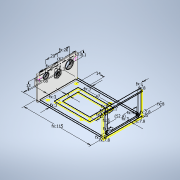
# Autodesk Inventor part: pi_shell_drill_guide_full
Saved by Autodesk Inventor 2022 (Build 260153000, 153)
## iProperties
Created: 2022-02-01
Part Number: pi_shell_drill_guide_full
Material: ABS Plastic
Document SubType Name: Modeling
Designer: Thomas
Density: 1.06 g/cm^3
Appearance: Smooth - White
Mass: 54.3446 g
Surface Area: 390.834 cm^2
Volume: 51.2684 cm^3
wall_thickness: 3.000 mm
outer_radius: 2.000 mm
inner_height: 38.000 mm
door_flange_thickness: 5.000 mm
m2p5_insert_top_diameter: 4.200 mm
insert_hole_angle: 8.00 deg
outer_width: 68.000 mm
outer_length: 115.000 mm
pcb_slide_thickness: 1.900 mm
Author: Thomas
Autodesk Inventor part; units mm, degrees
sketch "pi_base_plane" plane through (0, 0, 0) normal (0, 1, 0) x (-1, 0, 0)
  line L0 (0, 0) -> (115, 0)
  line L1 (115, 0) -> (115, 68)
  line L2 (115, 68) -> (0, 68)
  line L3 (0, 68) -> (0, 0)
  line L4 (3, 65) -> (112, 65)
  line L5 (112, 65) -> (112, 3)
  line L6 (112, 3) -> (3, 3)
  line L7 (3, 3) -> (3, 65)
  dimension "d0" = 115
  dimension "d1" = 68
  dimension "d2" = 3
  dimension "d3" = 3
  dimension "d4" = 3
  dimension "d5" = 3
  constraints: 16 end point, 4 parallel, 2 horizontal, 2 perpendicular
  measures "d0" distance of L2.end L1.end
  measures "d1" distance of L1.end L0.end
  measures "d2" distance between parallel lines of L4 L2
  measures "d3" distance between parallel lines of L1 L5
  measures "d4" distance between parallel lines of L0 L6
  measures "d5" distance between parallel lines of L3 L7
extrude "Extrusion1" add sketch "pi_base_plane" against normal blind 3 contours L3 L2 L1 L0 | L4 L5 L6 L7
extrude "Extrusion2" add sketch "pi_base_plane" along normal blind 38
sketch "pi_outline" plane through (0, 0, 0) normal (0, 1, 0) x (1, 0, 0)
  line L0 (-108, -6) -> (-23, -6)
  line L1 (-23, -6) -> (-23, -62)
  line L2 (-23, -62) -> (-108, -62)
  line L3 (-108, -62) -> (-108, -6)
  circle A0 centre (-104.5, -9.5) radius 1.35
  circle A1 centre (-104.5, -58.5) radius 1.35
  circle A2 centre (-46.5, -9.5) radius 1.35
  circle A3 centre (-46.5, -58.5) radius 1.35
  line L4 (-3, -65) -> (-112, -65) projected
  line L5 (-112, -3) -> (-3, -3) projected
  line L6 (-112, -65) -> (-112, -3) projected
  point P0 (0, 0)
  dimension "d10" = 56
  dimension "d11" = 85
  dimension "d12" = 2.7
  dimension "d13" = 3.5
  dimension "d14" = 3.5
  dimension "d15" = 2.7
  dimension "d16" = 3.5
  dimension "d17" = 3.5
  dimension "d18" = 2.7
  dimension "d19" = 3.5
  dimension "d20" = 58
  dimension "d21" = 2.7
  dimension "d22" = 3.5
  dimension "d23" = 58
  dimension "d24" = 62
  dimension "d25" = 3
  dimension "d26" = 4
  constraints: 8 end point, 4 centre point, 2 parallel, 1 horizontal, 1 perpendicular
  measures "d10" distance of L2.end L0.start
  measures "d11" distance between parallel lines of L1 L3
  measures "d12" diameter of A0
  measures "d13" distance from line of L0 A0.centre
  measures "d14" distance from line of A0.centre L3
  measures "d15" diameter of A1
  measures "d16" distance from line of L3 A1.centre
  measures "d17" distance from line of L2 A1.centre
  measures "d18" diameter of A2
  measures "d19" distance from line of A2.centre L0
  measures "d20" distance of A0.centre A2.centre
  measures "d21" diameter of A3
  measures "d22" distance from line of L2 A3.centre
  measures "d23" distance of A1.centre A3.centre
  measures "d24" distance between parallel lines of L4 L5
  measures "d25" distance between parallel lines of L0 L5
  measures "d26" distance between parallel lines of L3 L6
sketch "Sketch4" plane through (0, 0, 0) normal (0, 1, 0) x (1, 0, 0)
  circle A0 centre (-104.5, -9.5) radius 3.25
  circle A1 centre (-46.5, -9.5) radius 3.25
  circle A2 centre (-46.5, -58.5) radius 3.25
  circle A3 centre (-104.5, -58.5) radius 3.25
  point P0 (0, 0)
  dimension "d27" = 6.5
  dimension "d28" = 6.5
  dimension "d29" = 6.5
  dimension "d30" = 6.5
  constraints: 4 centre point, 4 coincident
  measures "d27" diameter of A0
  measures "d28" diameter of A3
  measures "d29" diameter of A1
  measures "d30" diameter of A2
extrude "Extrusion3" add sketch "Sketch4" along normal blind 0.4
sketch "Sketch5" plane through (-104.5, 0.4, 9.5) normal (0, 1, 0) x (1, 0, 0)
  circle A0 centre (0, 0) radius 3.25 projected
  circle A1 centre (0, 0) radius 2.1
  point P0 (104.5, 9.5)
  dimension "d34" = 4.2
  constraints: 1 centre point, 1 coincident
  measures "d34" diameter of A1
ref_plane "Work Plane1" through (-104.5, 0.4, 9.5) normal (0, 0, 1) x (1, 0, 0)
sketch "Sketch6" plane through (-104.5, 0.4, 9.5) normal (0, 0, 1) x (1, 0, 0)
  line L0 (3.25, 0) -> (-3.25, 0) projected
  line L1 (0, 0) -> (2.1, 0)
  line L2 (2.1, 0) -> (1.6222, -3.4)
  line L3 (-10.5, -3.4) -> (104.5, -3.4) projected
  line L4 (0, -3.4) -> (0, 0)
  line L5 (0, -3.4) -> (1.6222, -3.4)
  point P0 (104.5, -0.4)
  dimension "d35" = 2.1
  dimension "d36" = 82
  constraints: 8 end point, 3 point on line, 1 collinear, 1 midpoint, 1 perpendicular
  measures "d35" distance of L1.start L1.end
  measures "d36" angle of L0 L2
revolve "Revolution1" cut sketch "Sketch6" angle 360 about axis through (-104.5, -3, 9.5) along (0, 1, 0)
pattern_sketch "Sketch Driven Pattern1" of "Revolution1" from (-104.5, 0, 9.5) copies at (-46.5, 0, 9.5) at (-46.5, 0, 58.5) at (-104.5, 0, 58.5)
sketch "door" plane through (0, -3, 68) normal (1, 0, 0) x (0, 0, -1)
  line L0 (0, 41) -> (68, 41) projected
  line L1 (8, 41) -> (60, 41)
  line L2 (60, 41) -> (60, 13)
  line L3 (55, 8) -> (13, 8)
  line L4 (8, 13) -> (8, 41)
  line L5 (0, 0) -> (0, 41) projected
  line L6 (68, 0) -> (0, 0) projected
  line L7 (68, 0) -> (68, 41) projected
  arc A0 (55, 8) -> (60, 13) centre (55, 13) ccw
  arc A1 (8, 13) -> (13, 8) centre (13, 13) ccw
  line L8 (3, 46) -> (65, 46)
  line L9 (65, 46) -> (65, 13)
  arc A2 (55, 3) -> (65, 13) centre (55, 13) ccw
  line L10 (55, 3) -> (13, 3)
  arc A3 (3, 13) -> (13, 3) centre (13, 13) ccw
  line L11 (3, 13) -> (3, 46)
  line L12 (3, 41) -> (65, 41)
  line L13 (1, 41) -> (67, 41)
  line L14 (67, 41) -> (67, 39.1)
  line L15 (67, 39.1) -> (1, 39.1)
  line L16 (1, 39.1) -> (1, 41)
  line L17 (3, 3) -> (3, 41) projected
  line L18 (65, 41) -> (3, 41) projected
  line L19 (3, 41) -> (65, 41)
  line L20 (65, 41) -> (65, 41)
  line L21 (65, 41) -> (3, 41)
  line L22 (3, 41) -> (3, 41)
  point P0 (68, 3)
  point P1 (3, 41)
  point P2 (65, 41)
  point P3 (3, 41)
  point P4 (65, 41)
  dimension "d38" = 8
  dimension "d39" = 8
  dimension "d40" = 8
  dimension "d41" = 5
  dimension "d42" = 5
  dimension "d62" = 1
  dimension "d63" = 1
  dimension "d64" = 0
  dimension "d65" = 1.9
  constraints: 34 end point, 8 point on circle, 7 parallel, 4 centre point, 4 perpendicular, 4 tangent, 3 horizontal, 3 point on line, 1 collinear, 1 equal radius, 5 other
  measures "d38" distance between parallel lines of L4 L5
  measures "d39" distance between parallel lines of L3 L6
  measures "d40" distance between parallel lines of L7 L2
  measures "d41" radius of A0
  measures "d42" distance between parallel lines of L4 L11
  measures "d62" distance between parallel lines of L5 L16
  measures "d63" distance between parallel lines of L7 L14
  measures "d64" distance between parallel lines of L13 L0
  measures "d65" distance between parallel lines of L13 L15
extrude "door_cut" cut sketch "door" against normal blind 3 contours L0 L2 L15 L4 | L15 L2 A0 L3 A1 L4
extrude "Extrusion5" cut sketch "door" against normal blind 2 contours L0 L4 L15 L11 | L15 L4 A1 L3 A0 L2 L9 A2 L10 A3 L11 | L0 L9 L15 L2
sketch "Sketch8" plane through (-2, -3, 68) normal (1, 0, 0) x (0, 0, -1)
  circle A0 centre (7.8, 7.8) radius 2.1
  line L0 (0, 0) -> (0, 41) projected
  line L1 (68, 0) -> (0, 0) projected
  circle A1 centre (60.2, 7.8) radius 2.1
  line L2 (68, 0) -> (68, 41) projected
  point P0 (68, 3)
  dimension "d47" = 4.2
  dimension "d48" = 7.8
  dimension "d49" = 7.8
  dimension "d50" = 4.2
  dimension "d51" = 7.8
  dimension "d52" = 7.8
  dimension "d57" = 52.4
  constraints: 2 centre point
  measures "d47" diameter of A0
  measures "d48" distance from line of L0 A0.centre
  measures "d49" distance from line of A0.centre L1
  measures "d50" diameter of A1
  measures "d51" distance from line of L2 A1.centre
  measures "d52" distance from line of L1 A1.centre
  measures "d57" distance of A1.centre A0.centre
ref_plane "Work Plane2" through (-2, 4.8, 60.2) normal (0, 0, 1) x (1, 0, 0)
sketch "Sketch10" plane through (-3, 0, 3) normal (-1, 0, 0) x (0, 0, 1)
  arc A0 (52, 5) -> (57, 10) centre (52, 10) ccw projected
  arc A1 (52, 0) -> (62, 10) centre (52, 10) ccw projected
  line L0 (52, 5) -> (52, 0)
  line L1 (52, 0) -> (62, 0)
  line L2 (62, 0) -> (62, 10)
  line L3 (62, 10) -> (57, 10)
  arc A2 (5, 10) -> (10, 5) centre (10, 10) ccw projected
  line L4 (10, 5) -> (10, 0)
  arc A3 (0, 10) -> (10, 0) centre (10, 10) ccw projected
  line L5 (5, 10) -> (0, 10)
  line L6 (0, 10) -> (0, 0)
  line L7 (10, 0) -> (52, 0) projected
  line L8 (0, 0) -> (10, 0)
  point P0 (-3, 0)
  point P1 (57, 10)
  constraints: 16 end point, 5 perpendicular, 3 tangent, 2 vertical, 1 horizontal
extrude "Extrusion6" add sketch "Sketch10" along normal blind 3
sketch "Sketch9" plane through (-2, 4.8, 60.2) normal (0, 0, 1) x (1, 0, 0)
  line L0 (0, 0) -> (0, -2.0969)
  line L1 (0, -2.1) -> (0, 2.1) projected
  line L2 (-4, 5.2) -> (-4, 0.2) projected
  line L3 (-4, 0.2) -> (-4, -4.8) projected
  line L4 (-4, 5.2) -> (-4, -4.8) projected
  line L5 (0, 0) -> (0, -2.1)
  line L6 (0, -2.1) -> (-4, -1.5378)
  line L7 (-4, 0) -> (0, 0)
  line L8 (-4, -1.5378) -> (-4, 0)
  line L9 (-4, 0.2) -> (-4, -4.8) projected
  point P0 (2, -4.8)
  point P1 (-4, 0)
  point P2 (-4, -1.5378)
  dimension "d55" = 82
  constraints: 10 end point, 2 collinear, 2 point on line, 1 perpendicular, 1 vertical
  measures "d55" angle of L6 L0
revolve "Revolution2" cut sketch "Sketch9" angle 360 about axis through (-6, 4.8, 60.2) along (1, 0, 0)
ref_plane "Work Plane3" through (-2, 4.8, 7.8) normal (0, 0, -1) x (-1, 0, 0)
sketch "Sketch11" plane through (-2, 4.8, 7.8) normal (0, 0, -1) x (-1, 0, 0)
  line L0 (0, 2.1) -> (0, -2.1) projected
  line L1 (4, -4.8) -> (4, 5.2) projected
  line L2 (4, -4.8) -> (4, 0.2) projected
  line L3 (4, 0.2) -> (4, 5.2) projected
  line L4 (0, 0) -> (0, -2.1)
  line L5 (0, -2.1) -> (4, -1.5378)
  line L6 (4, -1.5378) -> (4, 0)
  line L7 (4, 0) -> (0, 0)
  point P0 (-2, -4.8)
  point P1 (4, 0)
  point P2 (4, -1.5378)
  dimension "d58" = 82
  constraints: 8 end point, 2 point on line, 1 collinear, 1 perpendicular
  measures "d58" angle of L0 L5
revolve "Revolution3" cut sketch "Sketch11" angle 360 about axis through (-6, 4.8, 7.8) along (1, 0, 0)
fillet "Fillet1" radius 1 6 edges at (-6, 10, 62.5) (-6, 6.4645, 58.5355) (-6, 2.5, 55) (-6, 2.5, 13) (-6, 6.4645, 9.4645) (-6, 10, 5.5)
fillet "Fillet2" radius 1 4 edges at (-49.75, 0, 58.5) (-107.75, 0, 58.5) (-49.75, 0, 9.5) (-107.75, 0, 9.5)
extrude "Extrusion7" cut sketch "door" against normal up to surface (112 mm away) contours L0 L11 L15 L16 | L0 L4 L15 L11 | L0 L2 L15 L4 | L0 L9 L15 L2 | L14 L15 L9 L0
sketch "Sketch12" plane through (-115, -3, 68) normal (0, 0, 1) x (1, 0, 0)
  line L0 (115, 39.1) -> (3, 39.1) projected
  circle A0 centre (20, 33) radius 1.325
  circle A1 centre (100, 33) radius 1.325
  line L1 (0, 0) -> (0, 41) projected
  line L2 (0, 41) -> (115, 41) projected
  line L3 (20, 33) -> (100, 33)
  point P0 (115, 3)
  dimension "d70" = 2.65
  dimension "d71" = 2.65
  dimension "d72" = 20
  dimension "d73" = 80
  dimension "d75" = 8
  constraints: 2 centre point, 2 end point, 1 horizontal
  measures "d70" diameter of A0
  measures "d71" diameter of A1
  measures "d72" distance from line of L1 L3.start
  measures "d73" distance of L3.end L3.start
  measures "d75" distance between parallel lines of L3 L2
extrude "M2.5 Side Fastners" cut sketch "Sketch12" against normal through all
sketch "Sketch14" plane through (-112, 0, 65) normal (1, 0, 0) x (0, 0, -1)
  line L0 (0, 36.1) -> (62, 36.1)
  circle A0 centre (31, 23.1) radius 3.15
  circle A1 centre (11, 30.1) radius 4.5
  circle A2 centre (51, 27) radius 6.5
  line L1 (36.5, 19.9246) -> (31, 16.7491)
  line L2 (31, 16.7491) -> (25.5, 19.9246)
  line L3 (25.5, 19.9246) -> (25.5, 26.2754)
  line L4 (25.5, 26.2754) -> (31, 29.4509)
  line L5 (31, 29.4509) -> (36.5, 26.2754)
  line L6 (36.5, 26.2754) -> (36.5, 19.9246)
  point P0 (65, 0)
  point P1 (0, 31)
  point P2 (62, 31)
  dimension "d78" = 6.3
  dimension "d79" = 9
  dimension "d80" = 13
  dimension "d81" = 6
  dimension "d82" = 9.1
  dimension "d84" = 62
  dimension "d85" = 31
  dimension "d90" = 11
  dimension "d93" = 13
  dimension "d94" = 20
  dimension "d95" = 20
  constraints: 14 end point, 3 centre point, 1 coincident, 1 horizontal, 1 vertical, 13 other
  measures "d78" diameter of A0
  measures "d79" diameter of A1
  measures "d80" diameter of A2
  measures "d81" vertical distance of A1.centre L0.start
  measures "d82" vertical distance of A2.centre L0.end
  measures "d84" distance of L0.end L0.start
  measures "d85" horizontal distance of A0.centre L0.start
  measures "d90" distance between parallel lines of L6 L3
  measures "d93" vertical distance of L0.start A0.centre
  measures "d94" horizontal distance of A0.centre A1.centre
  measures "d95" horizontal distance of A2.centre A0.centre
extrude "Connector and Mount Holes" cut sketch "Sketch14" against normal through all contours A0 | A1 | A2
extrude "Captive M6 Nut Indent" cut sketch "Sketch14" against normal blind 2 contours L1 L2 L3 L4 L5 L6
sketch "Sketch15" plane through (-115, -3, 0) normal (-1, 0, 0) x (0, 0, 1)
  line L0 (63.25, 30.75) -> (65.75, 30.75)
  line L1 (65.75, 30.75) -> (65.75, 19.75)
  line L2 (65.75, 19.75) -> (63.25, 19.75)
  line L3 (63.25, 19.75) -> (63.25, 30.75)
  line L4 (2.25, 30.75) -> (4.75, 30.75)
  line L5 (4.75, 30.75) -> (4.75, 19.75)
  line L6 (4.75, 19.75) -> (2.25, 19.75)
  line L7 (2.25, 19.75) -> (2.25, 30.75)
  line L8 (68, 0) -> (68, 41) projected
  line L9 (0, 41) -> (0, 0) projected
  circle A0 centre (34, 26.1) radius 3.15 projected
  point P0 (0, 3)
  dimension "d96" = 68
  dimension "d97" = 58.5
  dimension "d98" = 2.5
  dimension "d99" = 2.5
  dimension "d100" = 2.25
  dimension "d101" = 11
  dimension "d102" = 11
  dimension "d103" = 6.3
  dimension "d104" = 4.65
  dimension "d105" = 4.65
  constraints: 16 end point, 4 parallel, 2 horizontal, 2 perpendicular, 1 point on line
  measures "d96" distance between parallel lines of L8 L9
  measures "d97" distance between parallel lines of L3 L5
  measures "d98" distance between parallel lines of L5 L7
  measures "d99" distance between parallel lines of L1 L3
  measures "d100" distance between parallel lines of L7 L9
  measures "d101" distance between parallel lines of L4 L6
  measures "d102" distance of L0.end L1.end
  measures "d103" diameter of A0
  measures "d104" distance from line of A0.centre L4
  measures "d105" distance from line of A0.centre L0
extrude "Extrusion12" add sketch "Sketch15" along normal blind 5 contours L0 L1 L2 L3 | L4 L5 L6 L7
fillet "Fillet3" radius 5 2 edges at (-115, 16.75, 3.5) (-115, 16.75, 64.5)
sketch "Sketch16" plane through (0, 0, 0) normal (0, 1, 0) x (1, 0, 0)
  line L0 (-90.5, -47.5) -> (-43.5, -47.5)
  line L1 (-43.5, -47.5) -> (-43.5, -20.5)
  line L2 (-43.5, -20.5) -> (-90.5, -20.5)
  line L3 (-90.5, -20.5) -> (-90.5, -47.5)
  circle A0 centre (-104.5, -58.5) radius 2.1 projected
  circle A1 centre (-104.5, -9.5) radius 2.1 projected
  circle A2 centre (-46.5, -9.5) radius 2.1 projected
  circle A3 centre (-46.5, -58.5) radius 2.1 projected
  line L4 (-97.5, -54.5) -> (-36.5, -54.5)
  line L5 (-36.5, -54.5) -> (-36.5, -13.5)
  line L6 (-36.5, -13.5) -> (-97.5, -13.5)
  line L7 (-97.5, -13.5) -> (-97.5, -54.5)
  point P0 (0, 0)
  dimension "d109" = 47
  dimension "d110" = 27
  dimension "d111" = 14
  dimension "d112" = 11
  dimension "d113" = 7
  constraints: 16 end point, 4 parallel, 2 perpendicular, 1 horizontal, 3 other
  measures "d109" distance of L2.end L1.end
  measures "d110" distance of L1.end L0.end
  measures "d111" distance from line of A1.centre L3
  measures "d112" distance from line of L2 A2.centre
  measures "d113" distance between parallel lines of L3 L7
extrude "Extrusion13" cut sketch "Sketch16" against normal through all contours L3 L2 L1 L0
extrude "Extrusion14" cut sketch "Sketch16" against normal blind 2 contours L3 L2 L1 L0 | L7 L6 L5 L4
sketch "Sketch17" plane through (0, -2, 0) normal (0, 1, 0) x (1, 0, 0)
  circle A0 centre (-92.5, -49.5) radius 1.575
  line L0 (-36.5, -54.5) -> (-97.5, -54.5) projected
  line L1 (-90.5, -47.5) -> (-43.5, -47.5) projected
  line L2 (-97.5, -54.5) -> (-97.5, -13.5) projected
  circle A1 centre (-92.5, -18.5) radius 1.575
  line L3 (-97.5, -13.5) -> (-36.5, -13.5) projected
  circle A2 centre (-41.5, -49.5) radius 1.575
  line L4 (-36.5, -13.5) -> (-36.5, -54.5) projected
  circle A3 centre (-41.5, -18.5) radius 1.575
  line L5 (-90.5, -20.5) -> (-90.5, -47.5) projected
  line L6 (-90.5, -47.5) -> (-43.5, -47.5) projected
  point P0 (0, 0)
  point P1 (-90.5, -34)
  point P2 (-67, -47.5)
  dimension "d118" = 3.15
  dimension "d119" = 7
  dimension "d122" = 3.15
  dimension "d125" = 3.15
  dimension "d128" = 3.15
  dimension "d147" = 31
  dimension "d148" = 31
  dimension "d149" = 51
  dimension "d150" = 0
  dimension "d151" = 15.5
  dimension "d152" = 25.5
  dimension "d153" = 6
  dimension "d154" = 37
  constraints: 4 centre point, 2 midpoint
  measures "d118" diameter of A0
  measures "d119" distance between parallel lines of L0 L1
  measures "d122" diameter of A1
  measures "d125" diameter of A2
  measures "d128" diameter of A3
  measures "d147" distance of A2.centre A3.centre
  measures "d148" distance of A1.centre A0.centre
  measures "d149" distance of A2.centre A0.centre
  measures "d150" vertical distance of A3.centre A1.centre
  measures "d151" vertical distance of point (-90.5, -34) A0.centre
  measures "d152" horizontal distance of point (-67, -47.5) A0.centre
extrude "Extrusion15" cut sketch "Sketch17" against normal through all contours A0 | A1 | A2 | A3
sketch "Sketch18" plane through (0, 38, 0) normal (0, 1, 0) x (1, 0, 0)
  line L0 (-112, -65) -> (-113.5, -65)
  line L1 (-113.5, -65) -> (-113.5, -3)
  line L2 (-113.5, -3) -> (-112, -3)
  line L3 (-112, -3) -> (-112, -65)
  point P0 (0, 0)
  dimension "d133" = 1.5
  constraints: 8 end point, 2 parallel, 1 horizontal, 1 perpendicular
  measures "d133" distance between parallel lines of L3 L1
extrude "Extrusion16" add sketch "Sketch18" along normal blind 1
fillet "Fillet4" radius 0.5 3 edges at (-113.5, 38.5, 65) (-113.5, 39, 34) (-113.5, 38.5, 3)
sketch "Sketch19" plane through (0, -2, 0) normal (0, 1, 0) x (1, 0, 0)
  circle A0 centre (-41.5, -49.5) radius 1.575 projected
  circle A1 centre (-92.5, -18.5) radius 1.575 projected
  circle A2 centre (-41.5, -18.5) radius 1.575 projected
  circle A3 centre (-92.5, -49.5) radius 1.575 projected
  line L0 (-90.5, -47.5) -> (-43.5, -47.5) projected
  line L1 (-90.5, -20.5) -> (-90.5, -47.5) projected
  line L2 (-43.5, -20.5) -> (-90.5, -20.5) projected
  line L3 (-43.5, -47.5) -> (-43.5, -20.5) projected
  line L4 (-36.5, -13.5) -> (-36.5, -54.5) projected
  line L5 (-97.5, -13.5) -> (-36.5, -13.5) projected
  line L6 (-97.5, -54.5) -> (-97.5, -13.5) projected
  line L7 (-36.5, -54.5) -> (-97.5, -54.5) projected
  circle A4 centre (-41.5, -49.5) radius 1.575 projected
  circle A5 centre (-41.5, -18.5) radius 1.575 projected
  circle A6 centre (-92.5, -18.5) radius 1.575 projected
  circle A7 centre (-92.5, -49.5) radius 1.575 projected
  point P0 (0, 0)
sketch "Sketch20" plane through (-112, 0, 3) normal (0, 0, 1) x (1, 0, 0)
  line L0 (109, 36.1) -> (0, 36.1) projected
  line L1 (11.5, 36.1) -> (22.5, 36.1)
  line L2 (22.5, 36.1) -> (22.5, 27.1)
  line L3 (18.5, 23.1) -> (15.5, 23.1)
  line L4 (11.5, 27.1) -> (11.5, 36.1)
  circle A0 centre (17, 30) radius 1.325 projected
  arc A1 (11.5, 27.1) -> (15.5, 23.1) centre (15.5, 27.1) ccw
  arc A2 (18.5, 23.1) -> (22.5, 27.1) centre (18.5, 27.1) ccw
  point P0 (112, 0)
  point P1 (22.5, 23.1)
  point P2 (11.5, 23.1)
  point P3 (22.5, 36.1)
  dimension "d137" = 11
  dimension "d138" = 5.5
  dimension "d139" = 13
  dimension "d140" = 4
  constraints: 8 end point, 5 point on line, 4 point on circle, 4 tangent, 2 centre point, 2 parallel, 1 equal radius, 1 horizontal, 1 perpendicular
  measures "d137" distance of point (22.5, 23.1) point (11.5, 23.1)
  measures "d138" distance from line of A0.centre L4
  measures "d139" distance of point (11.5, 23.1) L1.start
  measures "d140" radius of A1
extrude "Extrusion17" cut sketch "Sketch20" against normal blind 1.1
pattern_linear "Rectangular Pattern1" count 2 spacing 80 along (1, 0, 0) of "Extrusion17"
ref_plane "Work Plane4" through (-115, -3, 34) normal (0, 0, 1) x (1, 0, 0)
mirror "Mirror1" about plane through (-115, -3, 34) normal (0, 0, 1) of "Extrusion17", "Rectangular Pattern1"
fillet "Fillet5" radius 1 2 edges at (-112, 30.1, 58.5) (-112, 27, 20.5)
sketch "Sketch21" plane through (-2, -3, 68) normal (1, 0, 0) x (0, 0, -1)
  line L0 (13, 8) -> (55, 8) projected
  line L1 (55, 3) -> (13, 3) projected
  line L2 (23, 8) -> (48, 8)
  line L3 (48, 8) -> (48, 3)
  line L4 (48, 3) -> (23, 3)
  line L5 (23, 3) -> (23, 8)
  line L6 (60, 13) -> (60, 39.1) projected
  line L7 (3, 13) -> (3, 39.1) projected
  point P0 (68, 3)
  point P1 (48, 8)
  dimension "d155" = 57
  dimension "d156" = 25
  dimension "d157" = 20
  constraints: 8 end point, 2 parallel, 2 point on line, 1 horizontal, 1 perpendicular
  measures "d155" distance between parallel lines of L6 L7
  measures "d156" distance between parallel lines of L3 L5
  measures "d157" distance between parallel lines of L5 L7
extrude "Extrusion18" cut sketch "Sketch21" against normal blind 1.1
fillet "Fillet6" radius 2 4 edges at (-2.5, 0, 45) (-2.5, 5, 45) (-2.5, 5, 20) (-2.5, 0, 20)
sketch "Sketch22" plane through (0, 38, 0) normal (0, 1, 0) x (1, 0, 0)
  line L0 (-115, -68) -> (0, -68) projected
  line L1 (-112, -68) -> (0, -68)
  line L2 (0, -68) -> (0, 0)
  line L3 (0, 0) -> (-112, 0)
  line L4 (-112, 0) -> (-112, -68)
  line L5 (-112, -65) -> (-112, -3) projected
  dimension "d161" = 0
  constraints: 8 end point, 2 parallel, 1 horizontal, 1 perpendicular, 1 point on line
  measures "d161" distance between parallel lines of L5 L4
extrude "Extrusion19" cut sketch "Sketch22" against normal through all
sketch "Sketch23" plane through (-115, -3, 0) normal (-1, 0, 0) x (0, 0, 1)
  line L0 (9.4456, 18.254) -> (35.2425, 18.254) construction
  line L1 (35.2425, 18.254) -> (35.2425, 14.2279) construction
  line L2 (35.2425, 14.2279) -> (9.4456, 14.2279) construction
  line L3 (9.4456, 14.2279) -> (9.4456, 18.254) construction
  line L4 (9.3329, 12.9532) -> (23.9776, 12.9532) construction
  line L5 (23.9776, 12.9532) -> (23.9776, 9.7051) construction
  line L6 (23.9776, 9.7051) -> (9.3329, 9.7051) construction
  line L7 (9.3329, 9.7051) -> (9.3329, 12.9532) construction
  spline S0 degree 2 poles (12.1577, 16.5917) (12.1577, 16.1743) (11.8193, 15.5024) (11.5353, 15.3147) knots 0 0 0 1 2 2 2
  spline S1 degree 2 poles (11.5353, 15.3147) (11.3031, 15.169) (10.8264, 15.0702) (10.4559, 15.0702) knots 0 0 0 1 2 2 2
  line L8 (10.4559, 15.0702) -> (9.7544, 15.0702)
  line L9 (9.7544, 15.0702) -> (9.7544, 18.1182)
  line L10 (9.7544, 18.1182) -> (10.4485, 18.1182)
  spline S2 degree 2 poles (10.4485, 18.1182) (10.8783, 18.1182) (11.3673, 17.9897) (11.5402, 17.8761) knots 0 0 0 1 2 2 2
  spline S3 degree 2 poles (11.5402, 17.8761) (11.8342, 17.681) (12.1577, 17.0363) (12.1577, 16.5917) knots 0 0 0 1 2 2 2
  spline S4 degree 2 poles (11.7354, 16.5966) (11.7354, 16.9474) (11.5032, 17.4438) (11.2735, 17.5846) knots 0 0 0 1 2 2 2
  spline S5 degree 2 poles (11.2735, 17.5846) (11.1104, 17.681) (10.7424, 17.7674) (10.4682, 17.7674) knots 0 0 0 1 2 2 2
  line L11 (10.4682, 17.7674) -> (10.1595, 17.7674)
  line L12 (10.1595, 17.7674) -> (10.1595, 15.4209)
  line L13 (10.1595, 15.4209) -> (10.4682, 15.4209)
  spline S6 degree 2 poles (10.4682, 15.4209) (10.7375, 15.4209) (11.145, 15.5074) (11.3105, 15.6234) knots 0 0 0 1 2 2 2
  spline S7 degree 2 poles (11.3105, 15.6234) (11.5229, 15.7667) (11.7354, 16.2409) (11.7354, 16.5966) knots 0 0 0 1 2 2 2
  line L14 (13.7805, 16.9449) -> (13.7608, 16.9449)
  spline S8 degree 2 poles (13.7608, 16.9449) (13.7163, 16.9573) (13.62, 16.9622) (13.5533, 16.9622) knots 0 0 0 1 2 2 2
  spline S9 degree 2 poles (13.5533, 16.9622) (13.3977, 16.9622) (13.0914, 16.8263) (12.9531, 16.693) knots 0 0 0 1 2 2 2
  line L15 (12.9531, 16.693) -> (12.9531, 15.0702)
  line L16 (12.9531, 15.0702) -> (12.5677, 15.0702)
  line L17 (12.5677, 15.0702) -> (12.5677, 17.3574)
  line L18 (12.5677, 17.3574) -> (12.9531, 17.3574)
  line L19 (12.9531, 17.3574) -> (12.9531, 17.0165)
  spline S10 degree 2 poles (12.9531, 17.0165) (13.163, 17.2043) (13.4767, 17.3574) (13.6249, 17.3574) knots 0 0 0 1 2 2 2
  spline S11 degree 2 poles (13.6249, 17.3574) (13.6842, 17.3574) (13.7435, 17.3525) (13.7805, 17.345) knots 0 0 0 1 2 2 2
  line L20 (13.7805, 17.345) -> (13.7805, 16.9449)
  line L21 (14.4721, 15.0702) -> (14.0868, 15.0702)
  line L22 (14.0868, 15.0702) -> (14.0868, 17.3574)
  line L23 (14.0868, 17.3574) -> (14.4721, 17.3574)
  line L24 (14.4721, 17.3574) -> (14.4721, 15.0702)
  line L25 (14.4993, 17.7378) -> (14.0621, 17.7378)
  line L26 (14.0621, 17.7378) -> (14.0621, 18.1379)
  line L27 (14.0621, 18.1379) -> (14.4993, 18.1379)
  line L28 (14.4993, 18.1379) -> (14.4993, 17.7378)
  line L29 (15.4305, 15.0702) -> (15.0452, 15.0702)
  line L30 (15.0452, 15.0702) -> (15.0452, 18.254)
  line L31 (15.0452, 18.254) -> (15.4305, 18.254)
  line L32 (15.4305, 18.254) -> (15.4305, 15.0702)
  line L33 (16.3889, 15.0702) -> (16.0035, 15.0702)
  line L34 (16.0035, 15.0702) -> (16.0035, 18.254)
  line L35 (16.0035, 18.254) -> (16.3889, 18.254)
  line L36 (16.3889, 18.254) -> (16.3889, 15.0702)
  line L37 (19.0046, 15.0702) -> (19.0046, 17.7575)
  line L38 (19.0046, 17.7575) -> (17.982, 17.7575)
  line L39 (17.982, 17.7575) -> (17.982, 18.1182)
  line L40 (17.982, 18.1182) -> (20.4323, 18.1182)
  line L41 (20.4323, 18.1182) -> (20.4323, 17.7575)
  line L42 (20.4323, 17.7575) -> (19.4097, 17.7575)
  line L43 (19.4097, 17.7575) -> (19.4097, 15.0702)
  line L44 (19.4097, 15.0702) -> (19.0046, 15.0702)
  spline S12 degree 2 poles (21.7043, 15.0183) (21.156, 15.0183) (20.5533, 15.6333) (20.5533, 16.2014) knots 0 0 0 1 2 2 2
  spline S13 degree 2 poles (20.5533, 16.2014) (20.5533, 16.7597) (21.1387, 17.4216) (21.6105, 17.4216) knots 0 0 0 1 2 2 2
  spline S14 degree 2 poles (21.6105, 17.4216) (21.8229, 17.4216) (22.1514, 17.2981) (22.2724, 17.1672) knots 0 0 0 1 2 2 2
  spline S15 degree 2 poles (22.2724, 17.1672) (22.3959, 17.0363) (22.5269, 16.6584) (22.5269, 16.3842) knots 0 0 0 1 2 2 2
  line L45 (22.5269, 16.3842) -> (22.5269, 16.1743)
  line L46 (22.5269, 16.1743) -> (20.9436, 16.1743)
  spline S16 degree 2 poles (20.9436, 16.1743) (20.9436, 15.7766) (21.3437, 15.3542) (21.6994, 15.3542) knots 0 0 0 1 2 2 2
  spline S17 degree 2 poles (21.6994, 15.3542) (21.8254, 15.3542) (22.0699, 15.411) (22.1687, 15.4555) knots 0 0 0 1 2 2 2
  spline S18 degree 2 poles (22.1687, 15.4555) (22.2724, 15.5049) (22.4157, 15.5913) (22.4626, 15.6309) knots 0 0 0 1 2 2 2
  line L47 (22.4626, 15.6309) -> (22.4849, 15.6309)
  line L48 (22.4849, 15.6309) -> (22.4849, 15.211)
  spline S19 degree 2 poles (22.4849, 15.211) (22.4182, 15.1838) (22.2156, 15.1047) (22.1366, 15.0825) knots 0 0 0 1 2 2 2
  spline S20 degree 2 poles (22.1366, 15.0825) (22.0254, 15.0504) (21.8427, 15.0183) (21.7043, 15.0183) knots 0 0 0 1 2 2 2
  spline S21 degree 2 poles (22.1514, 16.4682) (22.1465, 16.6238) (22.0822, 16.851) (22.0205, 16.9276) knots 0 0 0 1 2 2 2
  spline S22 degree 2 poles (22.0205, 16.9276) (21.9538, 17.0141) (21.7439, 17.1055) (21.5882, 17.1055) knots 0 0 0 1 2 2 2
  spline S23 degree 2 poles (21.5882, 17.1055) (21.4351, 17.1055) (21.2202, 17.0141) (21.1313, 16.9251) knots 0 0 0 1 2 2 2
  spline S24 degree 2 poles (21.1313, 16.9251) (21.0448, 16.8338) (20.9559, 16.6139) (20.9436, 16.4682) knots 0 0 0 1 2 2 2
  line L49 (20.9436, 16.4682) -> (22.1514, 16.4682)
  line L50 (25.5106, 15.0702) -> (25.5106, 16.3941)
  spline S25 degree 2 poles (25.5106, 16.3941) (25.5106, 16.5522) (25.4859, 16.8214) (25.4464, 16.8955) knots 0 0 0 1 2 2 2
  spline S26 degree 2 poles (25.4464, 16.8955) (25.4069, 16.977) (25.2562, 17.0561) (25.1253, 17.0561) knots 0 0 0 1 2 2 2
  spline S27 degree 2 poles (25.1253, 17.0561) (25.0067, 17.0561) (24.735, 16.9103) (24.5918, 16.772) knots 0 0 0 1 2 2 2
  spline S28 degree 2 poles (24.5918, 16.772) (24.5943, 16.7374) (24.5992, 16.6411) (24.5992, 16.5769) knots 0 0 0 1 2 2 2
  line L51 (24.5992, 16.5769) -> (24.5992, 15.0702)
  line L52 (24.5992, 15.0702) -> (24.2139, 15.0702)
  line L53 (24.2139, 15.0702) -> (24.2139, 16.3941)
  spline S29 degree 2 poles (24.2139, 16.3941) (24.2139, 16.5522) (24.1892, 16.8214) (24.1497, 16.8955) knots 0 0 0 1 2 2 2
  spline S30 degree 2 poles (24.1497, 16.8955) (24.1101, 16.977) (23.9595, 17.0561) (23.8285, 17.0561) knots 0 0 0 1 2 2 2
  spline S31 degree 2 poles (23.8285, 17.0561) (23.705, 17.0561) (23.4309, 16.9004) (23.3024, 16.7794) knots 0 0 0 1 2 2 2
  line L54 (23.3024, 16.7794) -> (23.3024, 15.0702)
  line L55 (23.3024, 15.0702) -> (22.9171, 15.0702)
  line L56 (22.9171, 15.0702) -> (22.9171, 17.3574)
  line L57 (22.9171, 17.3574) -> (23.3024, 17.3574)
  line L58 (23.3024, 17.3574) -> (23.3024, 17.1055)
  spline S32 degree 2 poles (23.3024, 17.1055) (23.4531, 17.2561) (23.7495, 17.4216) (23.9274, 17.4216) knots 0 0 0 1 2 2 2
  spline S33 degree 2 poles (23.9274, 17.4216) (24.1299, 17.4216) (24.4436, 17.2364) (24.5251, 17.0264) knots 0 0 0 1 2 2 2
  spline S34 degree 2 poles (24.5251, 17.0264) (24.7005, 17.2215) (25.0314, 17.4216) (25.2241, 17.4216) knots 0 0 0 1 2 2 2
  spline S35 degree 2 poles (25.2241, 17.4216) (25.3723, 17.4216) (25.6144, 17.3302) (25.7033, 17.2265) knots 0 0 0 1 2 2 2
  spline S36 degree 2 poles (25.7033, 17.2265) (25.7947, 17.1227) (25.896, 16.8115) (25.896, 16.5769) knots 0 0 0 1 2 2 2
  line L59 (25.896, 16.5769) -> (25.896, 15.0702)
  line L60 (25.896, 15.0702) -> (25.5106, 15.0702)
  spline S37 degree 2 poles (28.3536, 16.2755) (28.3536, 15.7025) (27.8077, 15.0257) (27.3903, 15.0257) knots 0 0 0 1 2 2 2
  spline S38 degree 2 poles (27.3903, 15.0257) (27.2199, 15.0257) (26.9581, 15.1047) (26.8222, 15.1863) knots 0 0 0 1 2 2 2
  line L61 (26.8222, 15.1863) -> (26.8222, 14.2279)
  line L62 (26.8222, 14.2279) -> (26.4369, 14.2279)
  line L63 (26.4369, 14.2279) -> (26.4369, 17.3574)
  line L64 (26.4369, 17.3574) -> (26.8222, 17.3574)
  line L65 (26.8222, 17.3574) -> (26.8222, 17.1178)
  spline S39 degree 2 poles (26.8222, 17.1178) (26.9655, 17.2487) (27.3162, 17.4216) (27.5212, 17.4216) knots 0 0 0 1 2 2 2
  spline S40 degree 2 poles (27.5212, 17.4216) (27.914, 17.4216) (28.3536, 16.7992) (28.3536, 16.2755) knots 0 0 0 1 2 2 2
  spline S41 degree 2 poles (27.9559, 16.2311) (27.9559, 16.6238) (27.7065, 17.0561) (27.4274, 17.0561) knots 0 0 0 1 2 2 2
  spline S42 degree 2 poles (27.4274, 17.0561) (27.2643, 17.0561) (26.9581, 16.9103) (26.8222, 16.7967) knots 0 0 0 1 2 2 2
  line L66 (26.8222, 16.7967) -> (26.8222, 15.4975)
  spline S43 degree 2 poles (26.8222, 15.4975) (26.9729, 15.4258) (27.1878, 15.3715) (27.3261, 15.3715) knots 0 0 0 1 2 2 2
  spline S44 degree 2 poles (27.3261, 15.3715) (27.625, 15.3715) (27.9559, 15.8112) (27.9559, 16.2311) knots 0 0 0 1 2 2 2
  line L67 (29.1465, 15.0702) -> (28.7612, 15.0702)
  line L68 (28.7612, 15.0702) -> (28.7612, 18.254)
  line L69 (28.7612, 18.254) -> (29.1465, 18.254)
  line L70 (29.1465, 18.254) -> (29.1465, 15.0702)
  spline S45 degree 2 poles (30.9867, 15.3122) (30.9397, 15.2776) (30.7816, 15.1541) (30.7075, 15.1171) knots 0 0 0 1 2 2 2
  spline S46 degree 2 poles (30.7075, 15.1171) (30.6063, 15.0628) (30.4161, 15.0059) (30.2432, 15.0059) knots 0 0 0 1 2 2 2
  spline S47 degree 2 poles (30.2432, 15.0059) (30.1024, 15.0059) (29.848, 15.1122) (29.7516, 15.2085) knots 0 0 0 1 2 2 2
  spline S48 degree 2 poles (29.7516, 15.2085) (29.6603, 15.3023) (29.5491, 15.579) (29.5491, 15.7321) knots 0 0 0 1 2 2 2
  spline S49 degree 2 poles (29.5491, 15.7321) (29.5491, 15.9692) (29.7492, 16.3052) (29.9665, 16.4015) knots 0 0 0 1 2 2 2
  spline S50 degree 2 poles (29.9665, 16.4015) (30.1592, 16.4904) (30.6828, 16.5571) (30.9867, 16.5744) knots 0 0 0 1 2 2 2
  line L71 (30.9867, 16.5744) -> (30.9867, 16.6485)
  spline S51 degree 2 poles (30.9867, 16.6485) (30.9867, 16.7819) (30.9051, 16.9474) (30.831, 16.9943) knots 0 0 0 1 2 2 2
  spline S52 degree 2 poles (30.831, 16.9943) (30.7569, 17.0412) (30.5445, 17.0709) (30.4309, 17.0709) knots 0 0 0 1 2 2 2
  spline S53 degree 2 poles (30.4309, 17.0709) (30.2975, 17.0709) (29.9369, 16.9918) (29.7566, 16.9153) knots 0 0 0 1 2 2 2
  line L72 (29.7566, 16.9153) -> (29.7344, 16.9153)
  line L73 (29.7344, 16.9153) -> (29.7344, 17.308)
  spline S54 degree 2 poles (29.7344, 17.308) (29.8406, 17.3376) (30.2382, 17.4117) (30.4334, 17.4117) knots 0 0 0 1 2 2 2
  spline S55 degree 2 poles (30.4334, 17.4117) (30.6705, 17.4117) (30.9941, 17.3376) (31.1225, 17.2413) knots 0 0 0 1 2 2 2
  spline S56 degree 2 poles (31.1225, 17.2413) (31.2485, 17.1474) (31.372, 16.8486) (31.372, 16.6337) knots 0 0 0 1 2 2 2
  line L74 (31.372, 16.6337) -> (31.372, 15.0702)
  line L75 (31.372, 15.0702) -> (30.9867, 15.0702)
  line L76 (30.9867, 15.0702) -> (30.9867, 15.3122)
  line L77 (30.9867, 15.6333) -> (30.9867, 16.2681)
  spline S57 degree 2 poles (30.9867, 16.2681) (30.8483, 16.2558) (30.4309, 16.2138) (30.3, 16.1743) knots 0 0 0 1 2 2 2
  spline S58 degree 2 poles (30.3, 16.1743) (30.1469, 16.1273) (29.9468, 15.9322) (29.9468, 15.7593) knots 0 0 0 1 2 2 2
  spline S59 degree 2 poles (29.9468, 15.7593) (29.9468, 15.5617) (30.1691, 15.3616) (30.3815, 15.3616) knots 0 0 0 1 2 2 2
  spline S60 degree 2 poles (30.3815, 15.3616) (30.5618, 15.3616) (30.8582, 15.5172) (30.9867, 15.6333) knots 0 0 0 1 2 2 2
  spline S61 degree 2 poles (32.6045, 15.0257) (32.2908, 15.0257) (31.9376, 15.3839) (31.9376, 15.7716) knots 0 0 0 1 2 2 2
  line L78 (31.9376, 15.7716) -> (31.9376, 17.0388)
  line L79 (31.9376, 17.0388) -> (31.6783, 17.0388)
  line L80 (31.6783, 17.0388) -> (31.6783, 17.3574)
  line L81 (31.6783, 17.3574) -> (31.9376, 17.3574)
  line L82 (31.9376, 17.3574) -> (31.9376, 18.0144)
  line L83 (31.9376, 18.0144) -> (32.3229, 18.0144)
  line L84 (32.3229, 18.0144) -> (32.3229, 17.3574)
  line L85 (32.3229, 17.3574) -> (33.0318, 17.3574)
  line L86 (33.0318, 17.3574) -> (33.0318, 17.0388)
  line L87 (33.0318, 17.0388) -> (32.3229, 17.0388)
  line L88 (32.3229, 17.0388) -> (32.3229, 15.9495)
  spline S62 degree 2 poles (32.3229, 15.9495) (32.3229, 15.7766) (32.3353, 15.5864) (32.3773, 15.5049) knots 0 0 0 1 2 2 2
  spline S63 degree 2 poles (32.3773, 15.5049) (32.4119, 15.4333) (32.5675, 15.3616) (32.7008, 15.3616) knots 0 0 0 1 2 2 2
  spline S64 degree 2 poles (32.7008, 15.3616) (32.7947, 15.3616) (32.9701, 15.4184) (33.0096, 15.4357) knots 0 0 0 1 2 2 2
  line L89 (33.0096, 15.4357) -> (33.0318, 15.4357)
  line L90 (33.0318, 15.4357) -> (33.0318, 15.0899)
  spline S65 degree 2 poles (33.0318, 15.0899) (32.9231, 15.0603) (32.7008, 15.0257) (32.6045, 15.0257) knots 0 0 0 1 2 2 2
  spline S66 degree 2 poles (34.3088, 15.0183) (33.7605, 15.0183) (33.1578, 15.6333) (33.1578, 16.2014) knots 0 0 0 1 2 2 2
  spline S67 degree 2 poles (33.1578, 16.2014) (33.1578, 16.7597) (33.7432, 17.4216) (34.215, 17.4216) knots 0 0 0 1 2 2 2
  spline S68 degree 2 poles (34.215, 17.4216) (34.4274, 17.4216) (34.7559, 17.2981) (34.8769, 17.1672) knots 0 0 0 1 2 2 2
  spline S69 degree 2 poles (34.8769, 17.1672) (35.0004, 17.0363) (35.1313, 16.6584) (35.1313, 16.3842) knots 0 0 0 1 2 2 2
  line L91 (35.1313, 16.3842) -> (35.1313, 16.1743)
  line L92 (35.1313, 16.1743) -> (33.5481, 16.1743)
  spline S70 degree 2 poles (33.5481, 16.1743) (33.5481, 15.7766) (33.9482, 15.3542) (34.3039, 15.3542) knots 0 0 0 1 2 2 2
  spline S71 degree 2 poles (34.3039, 15.3542) (34.4299, 15.3542) (34.6744, 15.411) (34.7732, 15.4555) knots 0 0 0 1 2 2 2
  spline S72 degree 2 poles (34.7732, 15.4555) (34.8769, 15.5049) (35.0202, 15.5913) (35.0671, 15.6309) knots 0 0 0 1 2 2 2
  line L93 (35.0671, 15.6309) -> (35.0894, 15.6309)
  line L94 (35.0894, 15.6309) -> (35.0894, 15.211)
  spline S73 degree 2 poles (35.0894, 15.211) (35.0227, 15.1838) (34.8201, 15.1047) (34.7411, 15.0825) knots 0 0 0 1 2 2 2
  spline S74 degree 2 poles (34.7411, 15.0825) (34.6299, 15.0504) (34.4471, 15.0183) (34.3088, 15.0183) knots 0 0 0 1 2 2 2
  spline S75 degree 2 poles (34.7559, 16.4682) (34.751, 16.6238) (34.6867, 16.851) (34.625, 16.9276) knots 0 0 0 1 2 2 2
  spline S76 degree 2 poles (34.625, 16.9276) (34.5583, 17.0141) (34.3483, 17.1055) (34.1927, 17.1055) knots 0 0 0 1 2 2 2
  spline S77 degree 2 poles (34.1927, 17.1055) (34.0396, 17.1055) (33.8247, 17.0141) (33.7358, 16.9251) knots 0 0 0 1 2 2 2
  spline S78 degree 2 poles (33.7358, 16.9251) (33.6493, 16.8338) (33.5604, 16.6139) (33.5481, 16.4682) knots 0 0 0 1 2 2 2
  line L95 (33.5481, 16.4682) -> (34.7559, 16.4682)
  line L96 (11.4645, 12.4567) -> (10.0467, 12.4567)
  line L97 (10.0467, 12.4567) -> (10.0467, 11.5971)
  line L98 (10.0467, 11.5971) -> (11.4052, 11.5971)
  line L99 (11.4052, 11.5971) -> (11.4052, 11.2365)
  line L100 (11.4052, 11.2365) -> (10.0467, 11.2365)
  line L101 (10.0467, 11.2365) -> (10.0467, 9.7693)
  line L102 (10.0467, 9.7693) -> (9.6416, 9.7693)
  line L103 (9.6416, 9.7693) -> (9.6416, 12.8173)
  line L104 (9.6416, 12.8173) -> (11.4645, 12.8173)
  line L105 (11.4645, 12.8173) -> (11.4645, 12.4567)
  line L106 (13.5763, 9.7693) -> (13.191, 9.7693)
  line L107 (13.191, 9.7693) -> (13.191, 10.0213)
  spline S79 degree 2 poles (13.191, 10.0213) (13.0132, 9.8657) (12.6946, 9.7051) (12.497, 9.7051) knots 0 0 0 1 2 2 2
  spline S80 degree 2 poles (12.497, 9.7051) (12.3488, 9.7051) (12.0845, 9.8039) (11.9881, 9.9101) knots 0 0 0 1 2 2 2
  spline S81 degree 2 poles (11.9881, 9.9101) (11.8893, 10.0163) (11.7806, 10.3399) (11.7806, 10.5721) knots 0 0 0 1 2 2 2
  line L108 (11.7806, 10.5721) -> (11.7806, 12.0566)
  line L109 (11.7806, 12.0566) -> (12.166, 12.0566)
  line L110 (12.166, 12.0566) -> (12.166, 10.7524)
  spline S82 degree 2 poles (12.166, 10.7524) (12.166, 10.5696) (12.1931, 10.33) (12.2401, 10.2411) knots 0 0 0 1 2 2 2
  spline S83 degree 2 poles (12.2401, 10.2411) (12.287, 10.1522) (12.4476, 10.0707) (12.5982, 10.0707) knots 0 0 0 1 2 2 2
  spline S84 degree 2 poles (12.5982, 10.0707) (12.739, 10.0707) (13.0576, 10.2312) (13.191, 10.3473) knots 0 0 0 1 2 2 2
  line L111 (13.191, 10.3473) -> (13.191, 12.0566)
  line L112 (13.191, 12.0566) -> (13.5763, 12.0566)
  line L113 (13.5763, 12.0566) -> (13.5763, 9.7693)
  line L114 (14.5273, 9.7693) -> (14.142, 9.7693)
  line L115 (14.142, 9.7693) -> (14.142, 12.9532)
  line L116 (14.142, 12.9532) -> (14.5273, 12.9532)
  line L117 (14.5273, 12.9532) -> (14.5273, 9.7693)
  line L118 (15.4857, 9.7693) -> (15.1003, 9.7693)
  line L119 (15.1003, 9.7693) -> (15.1003, 12.9532)
  line L120 (15.1003, 12.9532) -> (15.4857, 12.9532)
  line L121 (15.4857, 12.9532) -> (15.4857, 9.7693)
  spline S85 degree 2 poles (17.9779, 9.715) (17.7482, 9.715) (17.3505, 9.8385) (17.2196, 9.9076) knots 0 0 0 1 2 2 2
  line L122 (17.2196, 9.9076) -> (17.2196, 10.3399)
  line L123 (17.2196, 10.3399) -> (17.2394, 10.3399)
  spline S86 degree 2 poles (17.2394, 10.3399) (17.2888, 10.3004) (17.4222, 10.2065) (17.5333, 10.1546) knots 0 0 0 1 2 2 2
  spline S87 degree 2 poles (17.5333, 10.1546) (17.6296, 10.1077) (17.8668, 10.0386) (17.9927, 10.0386) knots 0 0 0 1 2 2 2
  spline S88 degree 2 poles (17.9927, 10.0386) (18.0841, 10.0386) (18.2941, 10.0805) (18.3435, 10.1151) knots 0 0 0 1 2 2 2
  spline S89 degree 2 poles (18.3435, 10.1151) (18.4151, 10.1621) (18.4793, 10.2683) (18.4793, 10.3769) knots 0 0 0 1 2 2 2
  spline S90 degree 2 poles (18.4793, 10.3769) (18.4793, 10.5128) (18.3311, 10.6536) (18.1409, 10.7005) knots 0 0 0 1 2 2 2
  spline S91 degree 2 poles (18.1409, 10.7005) (18.0668, 10.7178) (17.8297, 10.7672) (17.7284, 10.7944) knots 0 0 0 1 2 2 2
  spline S92 degree 2 poles (17.7284, 10.7944) (17.4666, 10.8709) (17.2295, 11.1871) (17.2295, 11.4119) knots 0 0 0 1 2 2 2
  spline S93 degree 2 poles (17.2295, 11.4119) (17.2295, 11.7231) (17.6963, 12.1109) (18.0817, 12.1109) knots 0 0 0 1 2 2 2
  spline S94 degree 2 poles (18.0817, 12.1109) (18.2719, 12.1109) (18.6572, 12.017) (18.7881, 11.9454) knots 0 0 0 1 2 2 2
  line L124 (18.7881, 11.9454) -> (18.7881, 11.5329)
  line L125 (18.7881, 11.5329) -> (18.7683, 11.5329)
  spline S95 degree 2 poles (18.7683, 11.5329) (18.6201, 11.6515) (18.2595, 11.7873) (18.0742, 11.7873) knots 0 0 0 1 2 2 2
  spline S96 degree 2 poles (18.0742, 11.7873) (17.8841, 11.7873) (17.6222, 11.6268) (17.6222, 11.4662) knots 0 0 0 1 2 2 2
  spline S97 degree 2 poles (17.6222, 11.4662) (17.6222, 11.3205) (17.7778, 11.1797) (17.9507, 11.1352) knots 0 0 0 1 2 2 2
  spline S98 degree 2 poles (17.9507, 11.1352) (18.0347, 11.113) (18.2471, 11.0685) (18.3632, 11.0414) knots 0 0 0 1 2 2 2
  spline S99 degree 2 poles (18.3632, 11.0414) (18.6152, 10.9772) (18.8721, 10.6832) (18.8721, 10.4288) knots 0 0 0 1 2 2 2
  spline S100 degree 2 poles (18.8721, 10.4288) (18.8721, 10.2806) (18.756, 10.0188) (18.6424, 9.9225) knots 0 0 0 1 2 2 2
  spline S101 degree 2 poles (18.6424, 9.9225) (18.5213, 9.8212) (18.2126, 9.715) (17.9779, 9.715) knots 0 0 0 1 2 2 2
  line L126 (19.6229, 9.7693) -> (19.2376, 9.7693)
  line L127 (19.2376, 9.7693) -> (19.2376, 12.0566)
  line L128 (19.2376, 12.0566) -> (19.6229, 12.0566)
  line L129 (19.6229, 12.0566) -> (19.6229, 9.7693)
  line L130 (19.6501, 12.4369) -> (19.2129, 12.4369)
  line L131 (19.2129, 12.4369) -> (19.2129, 12.8371)
  line L132 (19.2129, 12.8371) -> (19.6501, 12.8371)
  line L133 (19.6501, 12.8371) -> (19.6501, 12.4369)
  line L134 (21.6904, 9.7693) -> (20.0107, 9.7693)
  line L135 (20.0107, 9.7693) -> (20.0107, 10.0558)
  line L136 (20.0107, 10.0558) -> (21.2062, 11.7404)
  line L137 (21.2062, 11.7404) -> (20.0601, 11.7404)
  line L138 (20.0601, 11.7404) -> (20.0601, 12.0566)
  line L139 (20.0601, 12.0566) -> (21.6681, 12.0566)
  line L140 (21.6681, 12.0566) -> (21.6681, 11.7824)
  line L141 (21.6681, 11.7824) -> (20.4677, 10.0929)
  line L142 (20.4677, 10.0929) -> (21.6904, 10.0929)
  line L143 (21.6904, 10.0929) -> (21.6904, 9.7693)
  spline S102 degree 2 poles (23.0439, 9.7175) (22.4956, 9.7175) (21.8929, 10.3325) (21.8929, 10.9006) knots 0 0 0 1 2 2 2
  spline S103 degree 2 poles (21.8929, 10.9006) (21.8929, 11.4588) (22.4783, 12.1208) (22.9501, 12.1208) knots 0 0 0 1 2 2 2
  spline S104 degree 2 poles (22.9501, 12.1208) (23.1625, 12.1208) (23.491, 11.9973) (23.612, 11.8664) knots 0 0 0 1 2 2 2
  spline S105 degree 2 poles (23.612, 11.8664) (23.7355, 11.7355) (23.8664, 11.3575) (23.8664, 11.0834) knots 0 0 0 1 2 2 2
  line L144 (23.8664, 11.0834) -> (23.8664, 10.8734)
  line L145 (23.8664, 10.8734) -> (22.2832, 10.8734)
  spline S106 degree 2 poles (22.2832, 10.8734) (22.2832, 10.4757) (22.6833, 10.0534) (23.039, 10.0534) knots 0 0 0 1 2 2 2
  spline S107 degree 2 poles (23.039, 10.0534) (23.165, 10.0534) (23.4095, 10.1102) (23.5083, 10.1546) knots 0 0 0 1 2 2 2
  spline S108 degree 2 poles (23.5083, 10.1546) (23.612, 10.204) (23.7553, 10.2905) (23.8022, 10.33) knots 0 0 0 1 2 2 2
  line L146 (23.8022, 10.33) -> (23.8244, 10.33)
  line L147 (23.8244, 10.33) -> (23.8244, 9.9101)
  spline S109 degree 2 poles (23.8244, 9.9101) (23.7578, 9.8829) (23.5552, 9.8039) (23.4762, 9.7817) knots 0 0 0 1 2 2 2
  spline S110 degree 2 poles (23.4762, 9.7817) (23.365, 9.7496) (23.1822, 9.7175) (23.0439, 9.7175) knots 0 0 0 1 2 2 2
  spline S111 degree 2 poles (23.491, 11.1674) (23.4861, 11.323) (23.4218, 11.5502) (23.3601, 11.6268) knots 0 0 0 1 2 2 2
  spline S112 degree 2 poles (23.3601, 11.6268) (23.2934, 11.7132) (23.0834, 11.8046) (22.9278, 11.8046) knots 0 0 0 1 2 2 2
  spline S113 degree 2 poles (22.9278, 11.8046) (22.7747, 11.8046) (22.5598, 11.7132) (22.4709, 11.6243) knots 0 0 0 1 2 2 2
  spline S114 degree 2 poles (22.4709, 11.6243) (22.3844, 11.5329) (22.2955, 11.3131) (22.2832, 11.1674) knots 0 0 0 1 2 2 2
  line L148 (22.2832, 11.1674) -> (23.491, 11.1674)
  point P0 (0, 3)
  constraints: 4 other
extrude "Extrusion20" cut sketch "Sketch23" against normal blind 1
equation "\"d0\" = outer_length"
equation "\"d1\" = outer_width"
equation "\"d2\" = wall_thickness"
equation "\"d3\" = wall_thickness"
equation "\"d4\" = wall_thickness"
equation "\"d5\" = wall_thickness"
equation "\"d6\" = wall_thickness"
equation "\"d8\" = inner_height"
equation "\"d15\" = d12"
equation "\"d16\" = d14"
equation "\"d17\" = d13"
equation "\"d18\" = d12"
equation "\"d19\" = d13"
equation "\"d21\" = d12"
equation "\"d22\" = d17"
equation "\"d23\" = d20"
equation "\"d25\" = -0.5 * d10 + 0.5 * d24"
equation "\"d28\" = d27"
equation "\"d29\" = d27"
equation "\"d30\" = d27"
equation "\"d35\" = 0.5 * m2p5_insert_top_diameter"
equation "\"d38\" = wall_thickness + door_flange_thickness"
equation "\"d39\" = d38"
equation "\"d40\" = d38"
equation "\"d42\" = door_flange_thickness"
equation "\"d63\" = d62"
equation "\"d65\" = pcb_slide_thickness"
equation "\"d43\" = wall_thickness"
equation "\"d47\" = m2p5_insert_top_diameter"
equation "\"d48\" = d49"
equation "\"d50\" = d47"
equation "\"d51\" = d48"
equation "\"d52\" = d49"
equation "\"d71\" = d70"
equation "\"d85\" = 0.5 * d84"
equation "\"d95\" = d94"
equation "\"d99\" = d98"
equation "\"d100\" = -d98 + 0.5 * d96 - 0.5 * d97"
equation "\"d102\" = d101"
equation "\"d122\" = d118"
equation "\"d125\" = d118"
equation "\"d128\" = d118"
equation "\"d151\" = 0.5 * d148"
equation "\"d152\" = 0.5 * d149"
equation "\"d133\" = 0.5 * wall_thickness"
equation "\"d138\" = 0.5 * d137"
equation "\"wall_thickness\" = 3"
equation "\"outer_radius\" = 2"
equation "\"inner_height\" = 38"
equation "\"door_flange_thickness\" = 5"
equation "\"m2p5_insert_top_diameter\" = 4.2"
equation "\"insert_hole_angle\" = 8deg"
equation "\"outer_width\" = 68"
equation "\"outer_length\" = 115"
equation "\"pcb_slide_thickness\" = 1.9"
body "Solid1"
